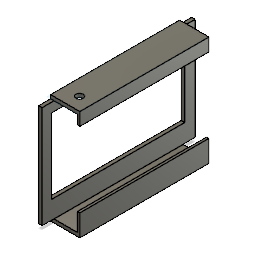
Vita Mount v1 (Autodesk Fusion 360 design; units mm, degrees)
Autodesk Fusion 360 part; units mm, degrees
sketch "Sketch1" plane through (0, 0, 0) normal (1, 0, 0) x (0, 0, -1)
  line L0 (0, 0) -> (182, 0)
  line L1 (182, 0) -> (182, 83.55)
  line L2 (182, 83.55) -> (0, 83.55)
  line L3 (0, 83.55) -> (0, 0)
  dimension "d1" = 83.55
  dimension "d2" = 182
  constraint horizontal L0
  constraint vertical L1
  constraint horizontal L2
  constraint vertical L3
  constraint coincident L0.start L3.end
  measures "d1" distance of L0.start L2.end
  measures "d2" distance of L0.start L0.end
extrude "Extrude1" add sketch "Sketch1" along normal blind 18.6 makes body 1
sketch "Sketch2" plane through (18.6, 0, 0) normal (1, 0, 0) x (0, 0, -1)
  line L0 (0, 83.55) -> (0, 0)
  line L1 (0, 0) -> (182, 0)
  line L2 (182, 0) -> (182, 83.55)
  line L3 (182, 83.55) -> (0, 83.55)
  line L4 (0, 41.775) -> (37, 41.775)
  line L5 (182, 41.775) -> (145, 41.775)
  line L6 (37, 41.775) -> (145, 41.775)
  line L7 (145, 41.775) -> (145, 83.55)
  line L8 (145, 83.55) -> (37, 83.55)
  line L9 (37, 83.55) -> (37, 41.775)
  line L10 (145, 41.775) -> (37, 41.775)
  line L11 (37, 41.775) -> (37, 0)
  line L12 (37, 0) -> (145, 0)
  line L13 (145, 0) -> (145, 41.775)
  arc A0 (145, 0) -> (145, 83.55) centre (139.9169, 41.775) ccw
  arc A1 (37, 83.55) -> (37, 0) centre (42.0831, 41.775) ccw
  dimension "d5" = 37
  dimension "d6" = 37
  constraint midpoint L0 L4.start
  constraint midpoint L2 L5.start
  constraint horizontal L6
  constraint vertical L7
  constraint horizontal L8
  constraint vertical L9
  constraint coincident L3 L7.end
  constraint horizontal L10
  constraint vertical L11
  constraint horizontal L12
  constraint vertical L13
  constraint coincident L1 L11.end
  constraint coincident L5.start A0
  constraint tangent L2 A0
  constraint coincident L4.start A1
  constraint tangent L0 A1
  measures "d5" distance of L4.start L4.end
  measures "d6" distance of L5.start L5.end
extrude "Extrude2" cut sketch "Sketch2" against normal blind 90 contours L0 L3 A1 | L0 L1 A1 | L2 L3 A0 | L1 L2 A0 bodies 1
sketch "Sketch3" plane through (18.6, 0, 0) normal (1, 0, 0) x (0, 0, -1)
  arc A0 (37, 83.55) -> (37, 0) centre (42.0831, 41.775) ccw
  line L0 (37, 0) -> (145, 0)
  arc A1 (145, 0) -> (145, 83.55) centre (139.9169, 41.775) ccw
  line L1 (145, 83.55) -> (37, 83.55)
  line L2 (145, 83.55) -> (193.2382, 83.55)
  line L3 (193.2382, 83.55) -> (193.2382, 74.55)
  line L4 (193.2382, 74.55) -> (145, 74.55)
  line L5 (145, 74.55) -> (145, 83.55)
  line L6 (37, 83.55) -> (-37.63, 83.55)
  line L7 (-37.63, 83.55) -> (-37.63, 74.55)
  line L8 (-37.63, 74.55) -> (37, 74.55)
  line L9 (37, 74.55) -> (37, 83.55)
  line L10 (37, 0) -> (-32.6872, 0)
  line L11 (-32.6872, 0) -> (-32.6872, 9)
  line L12 (-32.6872, 9) -> (37, 9)
  line L13 (37, 9) -> (37, 0)
  line L14 (145, 0) -> (203.1237, 0)
  line L15 (203.1237, 0) -> (203.1237, 9)
  line L16 (203.1237, 9) -> (145, 9)
  line L17 (145, 9) -> (145, 0)
  dimension "d9" = 9
  dimension "d10" = 9
  dimension "d11" = 9
  dimension "d12" = 9
  constraint horizontal L2
  constraint vertical L3
  constraint horizontal L4
  constraint vertical L5
  constraint coincident A1.end L1.start
  constraint horizontal L6
  constraint vertical L7
  constraint horizontal L8
  constraint vertical L9
  constraint coincident A0.start L1.end
  constraint horizontal L10
  constraint vertical L11
  constraint horizontal L12
  constraint vertical L13
  constraint coincident A0.end L0.start
  constraint horizontal L14
  constraint vertical L15
  constraint horizontal L16
  constraint vertical L17
  constraint coincident L0.end A1.start
  measures "d9" distance of A1.end L4.end
  measures "d10" distance of A0.start L8.end
  measures "d11" distance of A0.end L12.end
  measures "d12" distance of L0.end L16.end
extrude "Extrude3" cut sketch "Sketch3" against normal blind 6.25 contours A0 L8 L9 | A1 L4 L5 | A0 L12 L13 | A1 L16 L17 bodies 1
sketch "Sketch4" plane through (18.6, 0, 0) normal (1, 0, 0) x (0, 0, -1)
  line L0 (145, 74.55) -> (145, 83.55)
  line L1 (145, 83.55) -> (37, 83.55)
  line L2 (37, 83.55) -> (37, 74.55)
  line L3 (37, 74.55) -> (15.6864, 74.55)
  arc A0 (15.6864, 74.55) -> (15.6864, 9) centre (42.0831, 41.775) ccw
  line L4 (15.6864, 9) -> (37, 9)
  line L5 (37, 9) -> (37, 0)
  line L6 (37, 0) -> (145, 0)
  line L7 (145, 0) -> (145, 9)
  line L8 (145, 9) -> (166.3136, 9)
  arc A1 (166.3136, 9) -> (166.3136, 74.55) centre (139.9169, 41.775) ccw
  line L9 (166.3136, 74.55) -> (145, 74.55)
  line L10 (37, 83.55) -> (37, 84.55)
  line L11 (145, 83.55) -> (145, 84.55)
  line L12 (145, 84.55) -> (37, 84.55)
  line L13 (37, 84.55) -> (37, 87.55)
  line L14 (37, 87.55) -> (145, 87.55)
  line L15 (145, 87.55) -> (145, 84.55)
  dimension "d15" = 1
  dimension "d16" = 1
  dimension "d17" = 3
  constraint coincident L1.end L2.start
  constraint coincident L0.end L1.start
  constraint horizontal L12
  constraint vertical L13
  constraint horizontal L14
  constraint vertical L15
  measures "d15" distance of L1.end L10.end
  measures "d16" distance of L0.end L11.end
  measures "d17" distance of L11.end L14.end
extrude "Extrude4" add sketch "Sketch4" against normal blind 25 separate body contours L12 L13 L14 L15 makes body 2
sketch "Sketch5" plane through (18.6, 0, 0) normal (1, 0, 0) x (0, 0, -1)
  line L0 (145, 74.55) -> (145, 83.55)
  line L1 (145, 83.55) -> (37, 83.55)
  line L2 (37, 83.55) -> (37, 74.55)
  line L3 (37, 74.55) -> (15.6864, 74.55)
  arc A0 (15.6864, 74.55) -> (15.6864, 9) centre (42.0831, 41.775) ccw
  line L4 (15.6864, 9) -> (37, 9)
  line L5 (37, 9) -> (37, 0)
  line L6 (37, 0) -> (145, 0)
  line L7 (145, 0) -> (145, 9)
  line L8 (145, 9) -> (166.3136, 9)
  arc A1 (166.3136, 9) -> (166.3136, 74.55) centre (139.9169, 41.775) ccw
  line L9 (166.3136, 74.55) -> (145, 74.55)
  line L10 (0, 41.775) -> (35, 41.775)
  line L11 (35, 41.775) -> (40, 41.775)
  line L12 (40, 41.775) -> (40, 0)
  line L13 (40, 0) -> (35, 0)
  line L14 (35, 0) -> (35, 41.775)
  line L15 (37, 0) -> (35, 0)
  line L16 (35, 0) -> (35, 14.2)
  line L17 (35, 14.2) -> (37, 14.2)
  line L18 (37, 14.2) -> (37, 0)
  line L19 (35, 14.2) -> (146.25, 14.2)
  line L20 (146.25, 14.2) -> (146.25, 76.7)
  line L21 (146.25, 76.7) -> (35, 76.7)
  line L22 (35, 76.7) -> (35, 14.2)
  dimension "d20" = 35
  dimension "d21" = 14.2
  dimension "d22" = 111.25
  dimension "d23" = 62.5
  constraint midpoint A0 L10.start
  constraint horizontal L11
  constraint vertical L12
  constraint horizontal L13
  constraint vertical L14
  constraint coincident L6 L12.end
  constraint horizontal L15
  constraint vertical L16
  constraint horizontal L17
  constraint vertical L18
  constraint coincident L5.end L6.start
  constraint horizontal L19
  constraint vertical L20
  constraint horizontal L21
  constraint vertical L22
  measures "d20" distance of L10.start L10.end
  measures "d21" distance of L5.end L17.end
  measures "d22" distance of L16.end L19.end
  measures "d23" distance of L16.end L21.end
extrude "Extrude5" add 1 faces at (12.35, 80.1801, -35.0838) along direction (1, 0, 0) blind 6.25 on bodies 1 bodies 1
extrude "Extrude6" add 1 faces at (12.35, 80.1801, -146.9162) along direction (1, 0, 0) blind 6.25 on bodies 1 bodies 1
extrude "Extrude7" cut sketch "Sketch5" against normal blind 1 contours L0 L2 L3 L9 L11 L12 L19 L20 L21 L22 | L0 L9 L20 L21 | L2 L3 L21 L22 | L11 L12 L14 L17 L19 L22 bodies 1
sketch "Sketch6" plane through (0, 87.55, 0) normal (0, 1, 0) x (-1, 0, 0)
  line L0 (-18.6, -37) -> (-18.6, -145)
  line L1 (-18.6, -145) -> (6.4, -145)
  line L2 (6.4, -145) -> (6.4, -37)
  line L3 (6.4, -37) -> (-18.6, -37)
  line L4 (-10, -37) -> (-10, -45)
  circle A0 centre (-10, -48) radius 3
  dimension "d30" = 8
  dimension "d31" = 6
  constraint coincident L3 L4.start
  constraint coincident L4.end A0
  measures "d30" distance of L4.start L4.end
  measures "d31" diameter of A0
extrude "Extrude8" cut sketch "Sketch6" against normal blind 9 contours A0 bodies 2
sketch "Sketch7" plane through (0, 84.55, 0) normal (0, -1, 0) x (1, 0, 0)
  circle A0 centre (10, -48) radius 3
  line L0 (18.6, -145) -> (18.6, -37)
  line L1 (18.6, -37) -> (-6.4, -37)
  line L2 (-6.4, -37) -> (-6.4, -145)
  line L3 (-6.4, -145) -> (18.6, -145)
sketch "Sketch8" plane through (0, 0, 0) normal (0, -1, 0) x (1, 0, 0)
  line L0 (18.6, -37) -> (12.35, -37)
  line L1 (12.35, -37) -> (0, -37)
  line L2 (0, -37) -> (0, -145)
  line L3 (0, -145) -> (12.35, -145)
  line L4 (12.35, -145) -> (18.6, -145)
  line L5 (18.6, -145) -> (18.6, -37)
  line L6 (0, -145) -> (-0.5, -145)
  line L7 (-0.5, -145) -> (-6.4, -145)
  line L8 (-6.4, -145) -> (-6.4, -37)
  line L9 (-6.4, -37) -> (-0.5, -37)
  line L10 (-0.5, -37) -> (-0.5, -145)
  point P0 (-6.4, -37)
  dimension "d34" = 0.5
  constraint coincident L2.end L3.start
  constraint horizontal L7
  constraint vertical L8
  constraint horizontal L9
  constraint vertical L10
  constraint coincident P0 L8.end
  measures "d34" distance of L2.end L6.end
extrude "Extrude9" add sketch "Sketch8" against normal blind 85 contours L7 L8 L9 L10 bodies 2
extrude "Extrude10" cut 1 faces at (-6.4, 57.3667, -109) along direction (1, 0, 0) blind 2.9 on bodies 2 bodies 2
extrude "Extrude11" add 1 faces at (-1.5, 0, -109) along direction (0, -1, 0) blind 4 on bodies 2 bodies 2
sketch "Sketch9" plane through (-0.5, 0, 0) normal (1, 0, 0) x (0, 0, -1)
  line L0 (145, 84.55) -> (37, 84.55)
  line L1 (37, 84.55) -> (37, -4)
  line L2 (37, -4) -> (145, -4)
  line L3 (145, -4) -> (145, 84.55)
  line L4 (37, -4) -> (145, -4)
  line L5 (145, -4) -> (145, -1)
  line L6 (145, -1) -> (37, -1)
  line L7 (37, -1) -> (37, -4)
  constraint horizontal L4
  constraint vertical L5
  constraint horizontal L6
  constraint vertical L7
  constraint coincident L3 L5.end
  constraint coincident L1.end L2.start
extrude "Extrude12" add sketch "Sketch9" along normal blind 24 contours L1 L2 L3 L4 L5 L6 L7 bodies 2
extrude "Extrude13" add 1 faces at (18.6, 85.55, -73) along direction (1, 0, 0) blind 5 on bodies 2 bodies 2
sketch "Sketch10" plane through (0, -1, 0) normal (0, 1, 0) x (-1, 0, 0)
  line L0 (0.5, -145) -> (0.5, -37)
  line L1 (0.5, -37) -> (-23.5, -37)
  line L2 (-23.5, -37) -> (-23.5, -145)
  line L3 (-23.5, -145) -> (0.5, -145)
  line L4 (-23.5, -145) -> (-19.1, -145)
  line L5 (-19.1, -145) -> (-19.1, -37)
  line L6 (-19.1, -37) -> (-23.5, -37)
  line L7 (-23.5, -37) -> (-23.5, -145)
  dimension "d45" = 4.4
  constraint horizontal L4
  constraint vertical L5
  constraint horizontal L6
  constraint vertical L7
  constraint coincident L2.end L3.start
  measures "d45" distance of L2.end L4.end
extrude "Extrude14" add sketch "Sketch10" along normal blind 88 contours L1 L2 L3 L4 L5 L6 L7 bodies 2
extrude "Extrude15" cut 1 faces at (23.6, 85.55, -73) along direction (-1, 0, 0) blind 0.1 on bodies 2 bodies 2
sketch "Sketch11" plane through (23.5, 0, 0) normal (1, 0, 0) x (0, 0, -1)
  line L0 (37, 87.55) -> (37, -4)
  line L1 (37, -4) -> (145, -4)
  line L2 (145, -4) -> (145, 87.55)
  line L3 (145, 87.55) -> (37, 87.55)
  line L4 (37, 76.7) -> (145, 76.7)
  line L5 (145, 76.7) -> (145, 14.2)
  line L6 (145, 14.2) -> (37, 14.2)
  line L7 (37, 14.2) -> (37, 76.7)
  point P0 (37, 83.55)
  constraint horizontal L4
  constraint vertical L5
  constraint horizontal L6
  constraint vertical L7
  constraint coincident L2 L5.end
  constraint coincident L0 L4.start
extrude "Extrude16" cut sketch "Sketch11" against normal blind 20 contours L0 L2 L4 L5 L6 L7 bodies 2
extrude "Extrude17" cut 1 faces at (23.5, 79.3167, -109) along direction (-1, 0, 0) blind 2.4 on bodies 2 bodies 2
extrude "Extrude18" cut 1 faces at (23.5, 8.1333, -109) along direction (-1, 0, 0) blind 2.4 on bodies 2 bodies 2
sketch "Sketch12" plane through (0, 0, -37) normal (0, 0, 1) x (1, 0, 0)
  line L0 (21.1, -4) -> (21.1, 14.2)
  line L1 (21.1, 14.2) -> (19.1, 14.2)
  line L2 (19.1, 14.2) -> (19.1, -1)
  line L3 (19.1, -1) -> (-0.5, -1)
  line L4 (-0.5, -1) -> (-0.5, 84.55)
  line L5 (-0.5, 84.55) -> (19.1, 84.55)
  line L6 (19.1, 84.55) -> (19.1, 76.7)
  line L7 (19.1, 76.7) -> (21.1, 76.7)
  line L8 (21.1, 76.7) -> (21.1, 87.55)
  line L9 (21.1, 87.55) -> (-3.5, 87.55)
  line L10 (-3.5, 87.55) -> (-3.5, -4)
  line L11 (-3.5, -4) -> (21.1, -4)
  line L12 (-0.5, 84.55) -> (-3.5, 84.55)
  line L13 (-3.5, 84.55) -> (-3.5, -0.969)
  line L14 (-3.5, -0.969) -> (-0.5, -0.969)
  line L15 (-0.5, -0.969) -> (-0.5, 84.55)
  constraint horizontal L12
  constraint vertical L13
  constraint horizontal L14
  constraint vertical L15
  constraint coincident L10 L13.end
  constraint coincident L4.end L5.start
extrude "Extrude19" add sketch "Sketch12" along normal blind 10 contours L4 L10 L12 L13 L14 L15 bodies 2
sketch "Sketch13" plane through (0, 0, -145) normal (0, 0, -1) x (-1, 0, 0)
  line L0 (-21.1, 14.2) -> (-21.1, -4)
  line L1 (-21.1, -4) -> (3.5, -4)
  line L2 (3.5, -4) -> (3.5, 87.55)
  line L3 (3.5, 87.55) -> (-21.1, 87.55)
  line L4 (-21.1, 87.55) -> (-21.1, 76.7)
  line L5 (-21.1, 76.7) -> (-19.1, 76.7)
  line L6 (-19.1, 76.7) -> (-19.1, 84.55)
  line L7 (-19.1, 84.55) -> (0.5, 84.55)
  line L8 (0.5, 84.55) -> (0.5, -1)
  line L9 (0.5, -1) -> (-19.1, -1)
  line L10 (-19.1, -1) -> (-19.1, 14.2)
  line L11 (-19.1, 14.2) -> (-21.1, 14.2)
  line L12 (0, 84.55) -> (3.5, 84.55)
  line L13 (3.5, 84.55) -> (3.5, -0.969)
  line L14 (3.5, -0.969) -> (0, -0.969)
  line L15 (0, -0.969) -> (0, 84.55)
  point P0 (0, 84.55)
  point P1 (3.5, -0.969)
  constraint horizontal L12
  constraint vertical L13
  constraint horizontal L14
  constraint vertical L15
  constraint coincident P1 L13.end
  constraint coincident P0 L12.start
extrude "Extrude20" add sketch "Sketch13" along normal blind 10 contours L2 L8 L12 L13 L14 bodies 2
extrude "Extrude21" cut 1 faces at (17.6, 35.0333, -72.0833) along direction (-1, 0, 0) blind 71 on bodies 1 bodies 2
hidden bodies 1
named bodies: "Vita"
